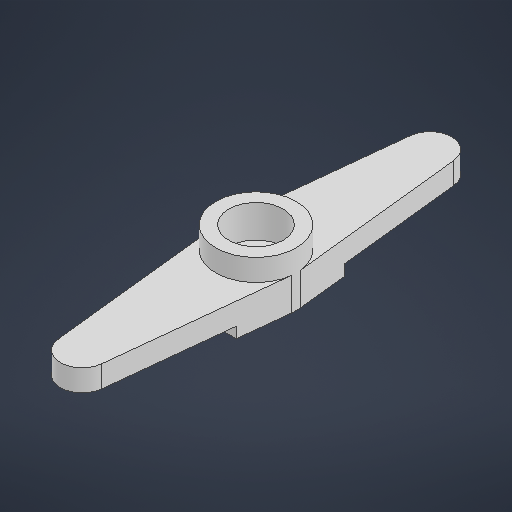
# Autodesk Inventor part: MG90s Arm
Saved by Autodesk Inventor 2025.1 (Build 291241000, 241)
## iProperties
Created: 2025-02-19
Part Number: MG90s Arm
Material: Generic
Document SubType Name: Modeling
Designer: jerem
Density: 1 g/cm^3
Appearance: Default
Author: jerem
Autodesk Inventor part; units mm, degrees
ref_plane "YZ Plane" through (0, 0, 0) normal (1, 0, 0) x (0, 1, 0)
ref_plane "XZ Plane" through (0, 0, 0) normal (0, 1, 0) x (-1, 0, 0)
ref_plane "XY Plane" through (0, 0, 0) normal (0, 0, 1) x (1, 0, 0)
sketch "Sketch1" plane through (0, 0, 0) normal (0, 1, 0) x (-1, 0, 0)
  circle A0 centre (0, 0) radius 3.7
  circle A1 centre (0, 16) radius 2
  line L0 (0, 16) -> (0, 0) construction
  line L1 (1.9887, 16.2125) -> (3.6791, 0.3931)
  line L2 (-3.6791, 0.3931) -> (-1.9887, 16.2125)
  line L3 (0, 16) -> (0, 18) construction
  line L4 (0, 0) -> (3.7, 0) construction
  circle A2 centre (0, -16) radius 2
  line L5 (0, -16) -> (0, 0) construction
  line L6 (1.9887, -16.2125) -> (3.6791, -0.3931)
  line L7 (-3.6791, -0.3931) -> (-1.9887, -16.2125)
  line L8 (0, -16) -> (0, -18) construction
  point P0 (3.6791, -0.3931)
  dimension "d0" = 4
  dimension "d1" = 7.4
  dimension "d2" = 18
  constraints: 18 end point, 9 point on circle, 6 symmetric about line, 4 tangent, 3 centre point, 2 point on line, 1 coincident, 1 horizontal, 1 vertical, 1 other
  measures "d0" diameter of A1
  measures "d1" diameter of A0
  measures "d2" distance of point (0, 0) L3.end
extrude "Extrusion1" add sketch "Sketch1" along normal blind 2
sketch "Sketch2" plane through (0, 2, 0) normal (0, 1, 0) x (1, 0, 0)
  circle A0 centre (0, 0) radius 3.7
  arc A1 (3.6791, -0.3931) -> (3.6791, 0.3931) centre (0, 0) ccw projected
  line L0 (3.6791, 0.3931) -> (1.9887, 16.2125) projected
  arc A2 (1.9887, 16.2125) -> (-1.9887, 16.2125) centre (0, 16) ccw projected
  line L1 (-1.9887, 16.2125) -> (-3.6791, 0.3931) projected
  arc A3 (-3.6791, 0.3931) -> (-3.6791, -0.3931) centre (0, 0) ccw projected
  line L2 (-3.6791, -0.3931) -> (-1.9887, -16.2125) projected
  arc A4 (-1.9887, -16.2125) -> (1.9887, -16.2125) centre (0, -16) ccw projected
  line L3 (1.9887, -16.2125) -> (3.6791, -0.3931) projected
  circle A5 centre (0, 0) radius 2.5
  point P0 (-3.7, 0)
  dimension "d5" = 1.2
  constraints: 2 coincident, 1 centre point, 1 horizontal alignment, 1 point on circle, 2 other
extrude "Extrusion2" add sketch "Sketch2" along normal blind 2 contours A0
extrude "Extrusion3" cut sketch "Sketch2" against normal blind 1 contours A5
sketch "Sketch3" plane through (0, 0, 0) normal (0, -1, 0) x (1, 0, 0)
  arc A0 (3.6791, -0.3931) -> (3.6791, 0.3931) centre (0, 0) ccw projected
  line L0 (1.9887, 16.2125) -> (3.6791, 0.3931) projected
  arc A1 (1.9887, 16.2125) -> (-1.9887, 16.2125) centre (0, 16) ccw projected
  line L1 (-3.6791, 0.3931) -> (-1.9887, 16.2125) projected
  arc A2 (-3.6791, 0.3931) -> (-3.6791, -0.3931) centre (0, 0) ccw projected
  line L2 (-1.9887, -16.2125) -> (-3.6791, -0.3931) projected
  arc A3 (-1.9887, -16.2125) -> (1.9887, -16.2125) centre (0, -16) ccw projected
  line L3 (3.6791, -0.3931) -> (1.9887, -16.2125) projected
  line L4 (3.1868, 5) -> (-3.1868, 5)
  line L5 (3.1868, -5) -> (-3.1868, -5)
  line L6 (0, 5) -> (0, -5) construction
  dimension "d10" = 10
  constraints: 6 end point, 4 point on line, 3 midpoint, 2 horizontal, 1 coincident, 1 perpendicular
  measures "d10" distance between parallel lines of L5 L4
extrude "Extrusion4" add sketch "Sketch3" along normal blind 1 contours L3 L5 L2 A2 L1 L4 L0 A0
sketch "Sketch4" plane through (0, 1, 0) normal (0, 1, 0) x (1, 0, 0)
  point P0 (0, 0)
  point P1 (0, 0)
  constraints: 1 coincident
hole "Hole1" at (0, 1, 0) direction (0, -1, 0) diameter 2.3 end through all
body "Solid1"
